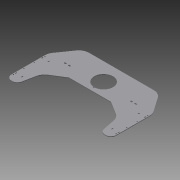
# Autodesk Inventor part: New shell2
Saved by Autodesk Inventor 2015 (Build 190159000, 159)
## iProperties
Created: 2011-09-21
Part Number: New shell2
Document SubType Name: Modeling
Designer: user
Density: 1 g/cm^3
Material: Generic
Appearance: Default
Author: user
Autodesk Inventor part; units mm, degrees
ref_plane "YZ Plane" through (0, 0, 0) normal (1, 0, 0) x (0, 1, 0)
ref_plane "XZ Plane" through (0, 0, 0) normal (0, 1, 0) x (-1, 0, 0)
ref_plane "XY Plane" through (0, 0, 0) normal (0, 0, 1) x (1, 0, 0)
sketch "Sketch44" plane through (0, 0, 0) normal (0, 1, 0) x (-1, 0, 0)
  line L0 (-100, 0) -> (-161.7026, -38.5641)
  line L1 (-250, -125) -> (-250, 34.2389)
  line L2 (-240.9616, 62.912) -> (-194.9288, 128.6731)
  line L3 (-153.9672, 150) -> (0, 150)
  line L4 (-195.9806, -129.9029) -> (-184.2316, -71.1582)
  line L5 (-220.4951, -150) -> (-225, -150)
  arc A0 (-161.7026, -38.5641) -> (-184.2316, -71.1582) centre (-135.2026, -80.964) ccw
  arc A1 (-240.9616, 62.912) -> (-250, 34.2389) centre (-200, 34.2389) ccw
  arc A2 (-153.9672, 150) -> (-194.9288, 128.6731) centre (-153.9672, 100) ccw
  arc A3 (-220.4951, -150) -> (-195.9806, -129.9029) centre (-220.4951, -125) ccw
  arc A4 (-250, -125) -> (-225, -150) centre (-225, -125) ccw
  circle A5 centre (-245, -120) radius 2.5
  circle A6 centre (-245, 30) radius 2.5
  line L6 (-163, 47) -> (-173, 47)
  line L7 (-173, 47) -> (-173, 53)
  line L8 (-173, 53) -> (-163, 53)
  line L9 (-163, 53) -> (-163, 47)
  line L10 (-244, -112) -> (-246, -112)
  line L11 (-247, -111) -> (-247, -105)
  line L12 (-246, -104) -> (-244, -104)
  line L13 (-243, -105) -> (-243, -111)
  line L14 (-214, -112) -> (-216, -112)
  line L15 (-217, -111) -> (-217, -105)
  line L16 (-216, -104) -> (-214, -104)
  line L17 (-213, -105) -> (-213, -111)
  arc A7 (-214, -112) -> (-213, -111) centre (-214, -111) ccw
  arc A8 (-217, -111) -> (-216, -112) centre (-216, -111) ccw
  arc A9 (-216, -104) -> (-217, -105) centre (-216, -105) ccw
  arc A10 (-213, -105) -> (-214, -104) centre (-214, -105) ccw
  arc A11 (-243, -105) -> (-244, -104) centre (-244, -105) ccw
  arc A12 (-246, -104) -> (-247, -105) centre (-246, -105) ccw
  arc A13 (-247, -111) -> (-246, -112) centre (-246, -111) ccw
  arc A14 (-244, -112) -> (-243, -111) centre (-244, -111) ccw
  line L18 (-244, 22) -> (-246, 22)
  line L19 (-247, 21) -> (-247, 15)
  line L20 (-246, 14) -> (-244, 14)
  line L21 (-243, 15) -> (-243, 21)
  line L22 (-214, 14) -> (-216, 14)
  line L23 (-217, 15) -> (-217, 21)
  line L24 (-216, 22) -> (-214, 22)
  line L25 (-213, 21) -> (-213, 15)
  arc A15 (-214, 14) -> (-213, 15) centre (-214, 15) ccw
  arc A16 (-217, 15) -> (-216, 14) centre (-216, 15) ccw
  arc A17 (-216, 22) -> (-217, 21) centre (-216, 21) ccw
  arc A18 (-213, 21) -> (-214, 22) centre (-214, 21) ccw
  arc A19 (-243, 21) -> (-244, 22) centre (-244, 21) ccw
  arc A20 (-246, 22) -> (-247, 21) centre (-246, 21) ccw
  arc A21 (-247, 15) -> (-246, 14) centre (-246, 15) ccw
  arc A22 (-244, 14) -> (-243, 15) centre (-244, 15) ccw
  line L26 (243, -105) -> (243, -111)
  arc A23 (243, -111) -> (244, -112) centre (244, -111) ccw
  arc A24 (184.2316, -71.1582) -> (161.7026, -38.5641) centre (135.2026, -80.964) ccw
  line L27 (100, 0) -> (161.7026, -38.5641)
  arc A25 (214, 22) -> (213, 21) centre (214, 21) ccw
  line L28 (216, 22) -> (214, 22)
  line L29 (213, 21) -> (213, 15)
  arc A26 (217, 21) -> (216, 22) centre (216, 21) ccw
  arc A27 (213, 15) -> (214, 14) centre (214, 15) ccw
  line L30 (214, 14) -> (216, 14)
  line L31 (217, 15) -> (217, 21)
  arc A28 (216, 14) -> (217, 15) centre (216, 15) ccw
  line L32 (217, -111) -> (217, -105)
  arc A29 (216, -112) -> (217, -111) centre (216, -111) ccw
  arc A30 (217, -105) -> (216, -104) centre (216, -105) ccw
  line L33 (214, -112) -> (216, -112)
  line L34 (216, -104) -> (214, -104)
  arc A31 (214, -104) -> (213, -105) centre (214, -105) ccw
  arc A32 (213, -111) -> (214, -112) centre (214, -111) ccw
  line L35 (213, -105) -> (213, -111)
  line L36 (173, 47) -> (173, 53)
  line L37 (163, 47) -> (173, 47)
  line L38 (163, 53) -> (163, 47)
  line L39 (173, 53) -> (163, 53)
  line L40 (240.9616, 62.912) -> (194.9288, 128.6731)
  arc A33 (194.9288, 128.6731) -> (153.9672, 150) centre (153.9672, 100) ccw
  line L41 (220.4951, -150) -> (225, -150)
  arc A34 (195.9806, -129.9029) -> (220.4951, -150) centre (220.4951, -125) ccw
  arc A35 (225, -150) -> (250, -125) centre (225, -125) ccw
  circle A36 centre (245, -120) radius 2.5
  line L42 (244, -112) -> (246, -112)
  line L43 (247, -111) -> (247, -105)
  arc A37 (246, -112) -> (247, -111) centre (246, -111) ccw
  line L44 (246, 14) -> (244, 14)
  arc A38 (243, 15) -> (244, 14) centre (244, 15) ccw
  arc A39 (246, 14) -> (247, 15) centre (246, 15) ccw
  line L45 (246, -104) -> (244, -104)
  arc A40 (244, -104) -> (243, -105) centre (244, -105) ccw
  arc A41 (247, -105) -> (246, -104) centre (246, -105) ccw
  line L46 (250, -125) -> (250, 34.2389)
  arc A42 (250, 34.2389) -> (240.9616, 62.912) centre (200, 34.2389) ccw
  circle A43 centre (245, 30) radius 2.5
  line L47 (247, 21) -> (247, 15)
  line L48 (243, 15) -> (243, 21)
  arc A44 (244, 22) -> (243, 21) centre (244, 21) ccw
  line L49 (244, 22) -> (246, 22)
  arc A45 (247, 21) -> (246, 22) centre (246, 21) ccw
  line L50 (153.9672, 150) -> (0, 150)
  line L51 (195.9806, -129.9029) -> (184.2316, -71.1582)
  arc A46 (4.7368, 20.25) -> (-4.7368, 20.25) centre (0, 65) ccw
  line L52 (-100, 0) -> (100, 0)
  line L53 (2.5, 17.7639) -> (2.5, 17.5)
  line L54 (0, 15) -> (0, 15)
  line L55 (-2.5, 17.5) -> (-2.5, 17.7639)
  arc A47 (-2.5, 17.7639) -> (-4.7368, 20.25) centre (-5, 17.7639) ccw
  arc A48 (-2.5, 17.5) -> (0, 15) centre (0, 17.5) ccw
  arc A49 (4.7368, 20.25) -> (2.5, 17.7639) centre (5, 17.7639) ccw
  arc A50 (0, 15) -> (2.5, 17.5) centre (0, 17.5) ccw
  circle A51 centre (-245, -70) radius 2.5
  circle A52 centre (245, -70) radius 2.5
  circle A53 centre (-245, -20) radius 2.5
  circle A54 centre (245, -20) radius 2.5
  line L56 (-153, 47) -> (-143, 47)
  line L57 (-143, 47) -> (-143, 53)
  line L58 (-143, 53) -> (-153, 53)
  line L59 (-153, 53) -> (-153, 47)
  line L60 (153, 47) -> (143, 47)
  line L61 (143, 47) -> (143, 53)
  line L62 (143, 53) -> (153, 53)
  line L63 (153, 53) -> (153, 47)
  line L64 (-100, -94.2682) -> (-100, 182.8574)
  line L65 (100, -80.964) -> (100, 178.1604)
  point P0 (0, 0)
  point P1 (0, 0)
  point P2 (-180, -50)
  point P3 (-250, -150)
  point P4 (-250, 50)
  point P5 (-180, 150)
  point P6 (-200, -150)
  point P7 (-243, -112)
  point P8 (-247, -104)
  point P9 (-247, -112)
  point P10 (-213, -112)
  point P11 (-217, -104)
  point P12 (-217, -112)
  point P13 (-247, 14)
  point P14 (-247, 22)
  point P15 (-243, 14)
  point P16 (-213, 14)
  point P17 (-217, 14)
  point P18 (-213, 22)
  point P19 (243, -112)
  point P20 (180, -50)
  point P21 (213, 22)
  point P22 (213, 14)
  point P23 (217, 14)
  point P24 (217, -112)
  point P25 (217, -104)
  point P26 (213, -112)
  point P27 (180, 150)
  point P28 (250, -150)
  point P29 (200, -150)
  point P30 (247, -104)
  point P31 (247, -112)
  point P32 (243, 14)
  point P33 (247, 14)
  point P34 (250, 50)
  point P35 (247, 22)
  point P36 (2.5, 15)
  point P37 (-2.5, 15)
  point P38 (-2.5, 20.0695)
  point P39 (2.5, 20.0695)
  dimension "d726" = 80
  dimension "d727" = 50
  dimension "d728" = 200
  dimension "d729" = 100
  dimension "d730" = 70
  dimension "d731" = 180
  dimension "d732" = 20
  dimension "d733" = 100
  dimension "d734" = 50
  dimension "d735" = 50
  dimension "d736" = 25
  dimension "d737" = 5
  dimension "d738" = 5
  dimension "d739" = 150
  dimension "d740" = 5
  dimension "d741" = 5
  dimension "d742" = 30
  dimension "d743" = 10
  dimension "d744" = 6
  dimension "d745" = 97
  dimension "d746" = 73
  dimension "d747" = 4
  dimension "d748" = 8
  dimension "d749" = 8
  dimension "d750" = 7
  dimension "d751" = 4
  dimension "d752" = 8
  dimension "d753" = 8
  dimension "d754" = 1
  dimension "d755" = 8
  dimension "d756" = 4
  dimension "d757" = 7
  dimension "d758" = 8
  dimension "d759" = 4
  dimension "d760" = 8
  dimension "d761" = 30
  dimension "d762" = 8
  dimension "d763" = 1
  dimension "d764" = 30
  dimension "d765" = 8
  dimension "d766" = 4
  dimension "d767" = 8
  dimension "d768" = 4
  dimension "d769" = 30
  dimension "d770" = 7
  dimension "d771" = 5
  dimension "d772" = 8
  dimension "d773" = 4
  dimension "d774" = 8
  dimension "d775" = 4
  dimension "d776" = 30
  dimension "d777" = 7
  dimension "d778" = 5
  dimension "d779" = 90
  dimension "d780" = 97
  dimension "d781" = 6
  dimension "d782" = 10
  dimension "d783" = 73
  dimension "d784" = 65
  dimension "d785" = 100
  dimension "d786" = 200
  dimension "d787" = 5
  dimension "d788" = 2.5
  dimension "d789" = 50
  constraints: 132 end point, 96 point on circle, 74 point on line, 55 centre point, 50 tangent, 20 equal radius, 17 parallel, 10 perpendicular, 7 horizontal
  measures "d726" horizontal distance of point (-180, -50) L0.start
  measures "d727" vertical distance of L0.start point (-180, -50)
  measures "d728" distance of point (-250, -150) point (-250, 50)
  measures "d729" vertical distance of point (-180, 150) point (-250, 50)
  measures "d730" horizontal distance of point (-250, 50) point (-180, 150)
  measures "d731" distance of point (-180, 150) L3.end
  measures "d732" horizontal distance of point (-200, -150) point (-180, -50)
  measures "d733" vertical distance of point (-200, -150) point (-180, -50)
  measures "d734" distance of point (-200, -150) point (-250, -150)
  measures "d735" radius of A0
  measures "d736" radius of A3
  measures "d737" diameter of A5
  measures "d738" diameter of A6
  measures "d739" distance of A6.centre A5.centre
  measures "d740" distance from line of L1 A5.centre
  measures "d741" distance from line of L1 A6.centre
  measures "d742" distance from line of L5 A5.centre
  measures "d743" distance of L8.start L8.end
  measures "d744" distance of L6.end L8.start
  measures "d745" distance between parallel lines of L3 L8
  measures "d746" distance from line of L0.start L7
  measures "d747" distance of point (-243, -112) point (-247, -112)
  measures "d748" distance of point (-247, -112) point (-247, -104)
  measures "d749" distance from line of L10 A5.centre
  measures "d750" distance between parallel lines of L1 L13
  measures "d751" distance of point (-213, -112) point (-217, -112)
  measures "d752" distance of point (-217, -112) point (-217, -104)
  measures "d753" distance from line of L14 A5.centre
  measures "d754" radius of A7
  measures "d755" distance of point (-247, 22) point (-247, 14)
  measures "d756" distance of point (-247, 14) point (-243, 14)
  measures "d757" distance between parallel lines of L1 L21
  measures "d758" distance from line of A6.centre L18
  measures "d759" distance of point (-213, 14) point (-217, 14)
  measures "d760" distance of point (-213, 22) point (-213, 14)
  measures "d761" distance between parallel lines of L19 L23
  measures "d762" distance from line of A6.centre L24
  measures "d763" radius of A15
  measures "d764" distance between parallel lines of L11 L15
  measures "d765" distance between parallel lines of L30 L28
  measures "d766" distance between parallel lines of L31 L29
  measures "d767" distance between parallel lines of L44 L49
  measures "d768" distance between parallel lines of L47 L48
  measures "d769" distance between parallel lines of L47 L31
  measures "d770" distance between parallel lines of L46 L48
  measures "d771" distance from line of L46 A43.centre
  measures "d772" distance between parallel lines of L33 L34
  measures "d773" distance between parallel lines of L32 L35
  measures "d774" distance between parallel lines of L42 L45
  measures "d775" distance between parallel lines of L43 L26
  measures "d776" distance between parallel lines of L43 L32
  measures "d777" distance between parallel lines of L46 L26
  measures "d778" distance from line of L46 A36.centre
  measures "d779" diameter of A46
  measures "d780" distance between parallel lines of L50 L39
  measures "d781" distance of L36.start L36.end
  measures "d782" distance of L37.start L36.start
  measures "d783" distance from line of L52.end L36
  measures "d784" distance from line of A46.centre L52
  measures "d785" distance of L0.start point (0, 0)
  measures "d786" distance of L0.start L52.end
  measures "d787" distance of point (2.5, 15) point (-2.5, 15)
  measures "d788" distance from line of A46.centre L55
  measures "d789" distance from line of A46.centre L54
extrude "Extrusion25" add sketch "Sketch44" along normal blind 3
body "Solid12"
